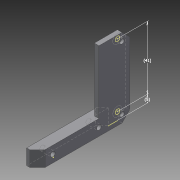
# Autodesk Inventor part: Z-stepper connector
Saved by Autodesk Inventor 2015 (Build 190159000, 159)
## iProperties
Created: 2019-01-12
Part Number: Z-stepper connector
Material: Generic
Document SubType Name: Modeling
Designer: Toby
Density: 1 g/cm^3
Appearance: Default
Author: Toby
Autodesk Inventor part; units mm, degrees
ref_plane "YZ Plane" through (0, 0, 0) normal (1, 0, 0) x (0, 1, 0)
ref_plane "XZ Plane" through (0, 0, 0) normal (0, 1, 0) x (-1, 0, 0)
ref_plane "XY Plane" through (0, 0, 0) normal (0, 0, 1) x (1, 0, 0)
sketch "Sketch1" plane through (0, 0, 0) normal (0, 0, 1) x (1, 0, 0)
  line L0 (-17.8598, 36.5888) -> (-10.8598, 36.5888)
  line L1 (-10.8598, 36.5888) -> (-10.8598, -13.4112)
  line L2 (-10.8598, -13.4112) -> (-17.8598, -13.4112)
  line L3 (-17.8598, -13.4112) -> (-17.8598, 36.5888)
  point P0 (0, 0)
  dimension "d0" = 7
  dimension "d1" = 50
  constraints: 8 end point, 2 parallel, 1 horizontal, 1 perpendicular
  measures "d0" distance between parallel lines of L1 L3
  measures "d1" distance between parallel lines of L2 L0
extrude "Extrusion1" add sketch "Sketch1" along normal blind 10
sketch "Sketch2" plane through (-17.8598, -13.4112, 0) normal (-1, 0, 0) x (0, 0, 1)
  line L0 (0, 0) -> (10, 0) projected
  line L1 (0, 50) -> (0, 0) projected
  point P0 (0, 13.4112)
  point P1 (5, 10)
  point P2 (5, 40)
  dimension "d4" = 10
  dimension "d5" = 5
  dimension "d6" = 5
  dimension "d7" = 30
  measures "d4" distance from line of L0 point (5, 10)
  measures "d5" distance from line of L1 point (5, 10)
  measures "d6" distance from line of L1 point (5, 40)
  measures "d7" distance of point (5, 10) point (5, 40)
hole "Hole1" at (-17.8598, -3.4112, 5) at (-17.8598, 26.5888, 5) direction (1, 0, 0) diameter 3 depth 7 tip angle 118
chamfer "Chamfer1" distance 5 angle 45 1 edges at (-10.8598, -13.4112, 5)
sketch "Sketch3" plane through (-17.8598, -13.4112, 0) normal (-1, 0, 0) x (0, 0, 1)
  line L0 (0, 50) -> (51, 50)
  line L1 (51, 50) -> (51, 60)
  line L2 (51, 60) -> (0, 60)
  line L3 (0, 60) -> (0, 50)
  line L4 (10, 50) -> (10, 0) projected
  line L5 (10, 40) -> (51, 40)
  line L6 (51, 40) -> (51, 50)
  line L7 (51, 50) -> (10, 50)
  line L8 (10, 50) -> (10, 40)
  point P0 (0, 13.4112)
  dimension "d18" = 51
  dimension "d19" = 10
  dimension "d20" = 10
  constraints: 16 end point, 4 parallel, 2 horizontal, 2 perpendicular, 1 point on line
  measures "d18" distance of L2.end L1.end
  measures "d19" distance of L1.end L0.end
  measures "d20" distance between parallel lines of L0 L5
extrude "Extrusion2" add sketch "Sketch3" against normal blind 7
sketch "Sketch4" plane through (-17.8598, -13.4112, 0) normal (-1, 0, 0) x (0, 0, 1)
  line L0 (0, 60) -> (51, 60) projected
  line L1 (51, 40) -> (10, 40)
  line L2 (10, 40) -> (10, 60)
  line L3 (10, 60) -> (51, 60)
  line L4 (51, 60) -> (51, 40)
  line L5 (10, 40) -> (10, 0) projected
  line L6 (0, 60) -> (0, 5) projected
  line L7 (10, 60) -> (0, 60)
  line L8 (0, 60) -> (0, 45)
  line L9 (0, 45) -> (10, 45)
  line L10 (10, 45) -> (10, 60)
  point P0 (0, 13.4112)
  dimension "d23" = 15
  constraints: 16 end point, 4 parallel, 2 horizontal, 2 perpendicular, 2 point on line, 1 collinear
  measures "d23" distance between parallel lines of L0 L9
extrude "Extrusion3" cut sketch "Sketch4" against normal blind 4
sketch "Sketch5" plane through (-13.8598, -13.4112, 0) normal (-1, 0, 0) x (0, 0, 1)
  line L0 (51, 60) -> (51, 40) projected
  line L1 (0, 45) -> (0, 60) projected
  line L2 (0, 60) -> (51, 60) projected
  point P0 (0, 13.4112)
  point P1 (5, 55)
  point P2 (46, 55)
  dimension "d26" = 5
  dimension "d27" = 5
  dimension "d28" = 5
  dimension "d29" = 5
  measures "d26" distance from line of L0 point (46, 55)
  measures "d27" distance from line of L1 point (5, 55)
  measures "d28" distance from line of L2 point (5, 55)
  measures "d29" distance from line of L2 point (46, 55)
hole "Hole2" at (-13.8598, 41.5888, 5) at (-13.8598, 41.5888, 46) direction (1, 0, 0) diameter 3 depth 7 tip angle 118 countersink diameter 6 countersink angle 90
chamfer "Chamfer2" distance 5 angle 45 2 edges at (-12.3598, 46.5888, 51) (-12.3598, 46.5888, 0)
chamfer "Chamfer3" distance 4 angle 45 1 edges at (-13.8598, 31.5888, 5)
sketch "Sketch6" plane through (-13.8598, -13.4112, 0) normal (-1, 0, 0) x (0, 0, 1)
  circle A0 centre (46, 55) radius 1.5 projected
  circle A1 centre (5, 55) radius 1.5 projected
  point P0 (0, 13.4112)
  dimension "d43" = 41
  constraints: 2 coincident
  measures "d43" distance of A1.centre point (46, 55)
sketch "Sketch7" plane through (-13.8598, -13.4112, 0) normal (-1, 0, 0) x (0, 0, 1)
  line L0 (0, 49) -> (0, 55) projected
  circle A0 centre (5, 55) radius 1.5 projected
  point P0 (0, 13.4112)
  dimension "d44" = 5
  measures "d44" distance from line of L0 A0.centre
body "Solid1"
